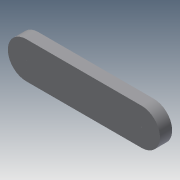
# Autodesk Inventor part: tahlo_sablona_servo
Saved by Autodesk Inventor 2013 (Build 170138000, 138)
## iProperties
Created: 2013-06-23
Part Number: tahlo_sablona_servo
Material: Generic
Document SubType Name: Modeling
Designer: idle-rug
Density: 1 g/cm^3
Author: idle-rug
Autodesk Inventor part; units mm, degrees
ref_plane "YZ Plane" through (0, 0, 0) normal (1, 0, 0) x (0, 1, 0)
ref_plane "XZ Plane" through (0, 0, 0) normal (0, 1, 0) x (-1, 0, 0)
ref_plane "XY Plane" through (0, 0, 0) normal (0, 0, 1) x (1, 0, 0)
sketch "Sketch1" plane through (0, 0, 0) normal (0, 1, 0) x (-1, 0, 0)
  line L0 (9.5, 3) -> (-9.5, 3)
  line L1 (-9.5, -3) -> (9.5, -3)
  circle A0 centre (-9.5, 0) radius 3
  circle A1 centre (9.5, 0) radius 3
  circle A2 centre (-9.5, 0) radius 0.05
  circle A3 centre (9.5, 0) radius 0.05
  line L2 (-9.5, 3) -> (9.5, 3)
  line L3 (-9.5, -3) -> (9.5, -3)
  arc A4 (-9.5, 3) -> (-9.5, -3) centre (-9.5, 0) ccw
  arc A5 (9.5, -3) -> (9.5, 3) centre (9.5, 0) ccw
  point P0 (0, 0)
  dimension "d0" = 19
  dimension "d1" = 6
  dimension "d2" = 0.1
  dimension "d3" = 0.1
  constraints: 8 end point, 4 centre point, 4 point on circle, 3 horizontal, 2 coincident, 2 parallel, 2 tangent, 2 vertical alignment, 5 other
  measures "d0" distance of L1.end L1.start
  measures "d1" distance of L1.start L0.end
  measures "d2" diameter of A2
  measures "d3" diameter of A3
extrude "Extrusion1" add sketch "Sketch1" along normal blind 2
body "Solid1"
